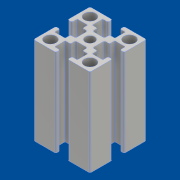
# Autodesk Inventor part: S31
Saved by Autodesk Inventor 2022.2 (Build 262287000, 287)
## iProperties
Created: 2018-10-03
Part Number: S31
Material: アルミニウム 6061
Document SubType Name: Modeling
Designer: gisen
Density: 2.7 g/cm^3
Appearance: アルミニウム - フラット
Author: gisen
Autodesk Inventor part; units mm, degrees
ref_plane "YZ Plane" through (0, 0, 0) normal (1, 0, 0) x (0, 1, 0)
ref_plane "XZ Plane" through (0, 0, 0) normal (0, 1, 0) x (-1, 0, 0)
ref_plane "XY Plane" through (0, 0, 0) normal (0, 0, 1) x (1, 0, 0)
sketch "BaseS" plane through (0, 0, 0) normal (0, 0, 1) x (1, 0, 0)
  line L0 (8.5, -3.8) -> (8.5, -2.6)
  line L1 (4, -8.3) -> (4, -5)
  circle A0 centre (7, -7) radius 2
  line L2 (10, -2.6) -> (10, -9.5)
  line L3 (2.6, -10) -> (9.5, -10)
  line L4 (2.1, -9.5) -> (2.1, -9)
  line L5 (8.5, -2.6) -> (8.5, -3.8)
  line L6 (3.8, -4.8) -> (2.6, -4.8)
  line L7 (4.8, -3.8) -> (4.8, -2.6)
  arc A1 (2.1, -4.3) -> (2.6, -4.8) centre (2.6, -4.3) ccw
  arc A2 (2.6, -8.5) -> (2.1, -9) centre (2.6, -9) ccw
  arc A3 (3.8, -8.5) -> (4, -8.3) centre (3.8, -8.3) ccw
  arc A4 (4, -5) -> (3.8, -4.8) centre (3.8, -5) ccw
  arc A5 (2.1, -3.5) -> (1.6, -3) centre (1.6, -3.5) ccw
  arc A6 (2.1, -9.5) -> (2.6, -10) centre (2.6, -9.5) ccw
  arc A7 (9.5, -10) -> (10, -9.5) centre (9.5, -9.5) ccw
  arc A8 (10, -2.6) -> (9.5, -2.1) centre (9.5, -2.6) ccw
  arc A9 (9, -2.1) -> (8.5, -2.6) centre (9, -2.6) ccw
  arc A10 (8.3, -4) -> (8.5, -3.8) centre (8.3, -3.8) ccw
  arc A11 (4.8, -3.8) -> (5, -4) centre (5, -3.8) ccw
  line L8 (4.3, -2.1) -> (3.5, -2.1)
  arc A12 (4.8, -2.6) -> (4.3, -2.1) centre (4.3, -2.6) ccw
  arc A13 (3, -1.6) -> (3.5, -2.1) centre (3.5, -1.6) ccw
  line L9 (2.1, -4.3) -> (2.1, -3.5)
  line L10 (3.8, -8.5) -> (2.6, -8.5)
  line L11 (9.5, -2.1) -> (9, -2.1)
  line L12 (8.3, -4) -> (5, -4)
  circle A14 centre (0, 0) radius 1.65
  arc A15 (8.5, 2.6) -> (9, 2.1) centre (9, 2.6) ccw
  line L13 (8.5, 3.8) -> (8.5, 2.6)
  arc A16 (8.5, 3.8) -> (8.3, 4) centre (8.3, 3.8) ccw
  line L14 (8.3, 4) -> (5, 4)
  line L15 (10, 2.6) -> (10, 9.5)
  arc A17 (10, 9.5) -> (9.5, 10) centre (9.5, 9.5) ccw
  circle A18 centre (7, 7) radius 2
  line L16 (4, 8.3) -> (4, 5)
  line L17 (2.6, 10) -> (9.5, 10)
  line L18 (9.5, 2.1) -> (9, 2.1)
  arc A19 (9.5, 2.1) -> (10, 2.6) centre (9.5, 2.6) ccw
  line L19 (3.8, 8.5) -> (2.6, 8.5)
  line L20 (4.8, 3.8) -> (4.8, 2.6)
  arc A20 (4.3, 2.1) -> (4.8, 2.6) centre (4.3, 2.6) ccw
  line L21 (2.6, 8.5) -> (3.8, 8.5)
  arc A21 (4, 8.3) -> (3.8, 8.5) centre (3.8, 8.3) ccw
  arc A22 (2.1, 9) -> (2.6, 8.5) centre (2.6, 9) ccw
  arc A23 (2.6, 10) -> (2.1, 9.5) centre (2.6, 9.5) ccw
  line L22 (2.1, 9.5) -> (2.1, 9)
  arc A24 (1.6, 3) -> (2.1, 3.5) centre (1.6, 3.5) ccw
  line L23 (3.8, 4.8) -> (2.6, 4.8)
  arc A25 (5, 4) -> (4.8, 3.8) centre (5, 3.8) ccw
  arc A26 (3.8, 4.8) -> (4, 5) centre (3.8, 5) ccw
  line L24 (4.3, 2.1) -> (3.5, 2.1)
  arc A27 (2.6, 4.8) -> (2.1, 4.3) centre (2.6, 4.3) ccw
  line L25 (2.1, 4.3) -> (2.1, 3.5)
  arc A28 (3.5, 2.1) -> (3, 1.6) centre (3.5, 1.6) ccw
  arc A29 (-2.6, 8.5) -> (-2.1, 9) centre (-2.6, 9) ccw
  line L26 (-3.8, 8.5) -> (-2.6, 8.5)
  arc A30 (-3.8, 8.5) -> (-4, 8.3) centre (-3.8, 8.3) ccw
  line L27 (-4, 8.3) -> (-4, 5)
  line L28 (-2.6, 10) -> (-9.5, 10)
  arc A31 (-9.5, 10) -> (-10, 9.5) centre (-9.5, 9.5) ccw
  circle A32 centre (-7, 7) radius 2
  line L29 (-8.3, 4) -> (-5, 4)
  line L30 (-10, 2.6) -> (-10, 9.5)
  line L31 (-2.1, 9.5) -> (-2.1, 9)
  arc A33 (-2.1, 9.5) -> (-2.6, 10) centre (-2.6, 9.5) ccw
  line L32 (-8.5, 3.8) -> (-8.5, 2.6)
  line L33 (-3.8, 4.8) -> (-2.6, 4.8)
  arc A34 (-2.1, 4.3) -> (-2.6, 4.8) centre (-2.6, 4.3) ccw
  line L34 (-8.5, 2.6) -> (-8.5, 3.8)
  arc A35 (-8.3, 4) -> (-8.5, 3.8) centre (-8.3, 3.8) ccw
  arc A36 (-9, 2.1) -> (-8.5, 2.6) centre (-9, 2.6) ccw
  arc A37 (-10, 2.6) -> (-9.5, 2.1) centre (-9.5, 2.6) ccw
  line L35 (-9.5, 2.1) -> (-9, 2.1)
  arc A38 (-3, 1.6) -> (-3.5, 2.1) centre (-3.5, 1.6) ccw
  line L36 (-4.8, 3.8) -> (-4.8, 2.6)
  arc A39 (-4, 5) -> (-3.8, 4.8) centre (-3.8, 5) ccw
  arc A40 (-4.8, 3.8) -> (-5, 4) centre (-5, 3.8) ccw
  line L37 (-2.1, 4.3) -> (-2.1, 3.5)
  arc A41 (-4.8, 2.6) -> (-4.3, 2.1) centre (-4.3, 2.6) ccw
  line L38 (-4.3, 2.1) -> (-3.5, 2.1)
  arc A42 (-2.1, 3.5) -> (-1.6, 3) centre (-1.6, 3.5) ccw
  arc A43 (-8.5, -2.6) -> (-9, -2.1) centre (-9, -2.6) ccw
  line L39 (-8.5, -3.8) -> (-8.5, -2.6)
  arc A44 (-8.5, -3.8) -> (-8.3, -4) centre (-8.3, -3.8) ccw
  line L40 (-8.3, -4) -> (-5, -4)
  line L41 (-10, -2.6) -> (-10, -9.5)
  arc A45 (-10, -9.5) -> (-9.5, -10) centre (-9.5, -9.5) ccw
  circle A46 centre (-7, -7) radius 2
  line L42 (-4, -8.3) -> (-4, -5)
  line L43 (-2.6, -10) -> (-9.5, -10)
  line L44 (-9.5, -2.1) -> (-9, -2.1)
  arc A47 (-9.5, -2.1) -> (-10, -2.6) centre (-9.5, -2.6) ccw
  line L45 (-3.8, -8.5) -> (-2.6, -8.5)
  line L46 (-4.8, -3.8) -> (-4.8, -2.6)
  arc A48 (-4.3, -2.1) -> (-4.8, -2.6) centre (-4.3, -2.6) ccw
  line L47 (-2.6, -8.5) -> (-3.8, -8.5)
  arc A49 (-4, -8.3) -> (-3.8, -8.5) centre (-3.8, -8.3) ccw
  arc A50 (-2.1, -9) -> (-2.6, -8.5) centre (-2.6, -9) ccw
  arc A51 (-2.6, -10) -> (-2.1, -9.5) centre (-2.6, -9.5) ccw
  line L48 (-2.1, -9.5) -> (-2.1, -9)
  arc A52 (-1.6, -3) -> (-2.1, -3.5) centre (-1.6, -3.5) ccw
  line L49 (-3.8, -4.8) -> (-2.6, -4.8)
  arc A53 (-5, -4) -> (-4.8, -3.8) centre (-5, -3.8) ccw
  arc A54 (-3.8, -4.8) -> (-4, -5) centre (-3.8, -5) ccw
  line L50 (-4.3, -2.1) -> (-3.5, -2.1)
  arc A55 (-2.6, -4.8) -> (-2.1, -4.3) centre (-2.6, -4.3) ccw
  line L51 (-2.1, -4.3) -> (-2.1, -3.5)
  arc A56 (-3.5, -2.1) -> (-3, -1.6) centre (-3.5, -1.6) ccw
  line L52 (1.6, -3) -> (-1.6, -3)
  line L53 (-3, -1.6) -> (-3, 1.6)
  line L54 (-1.6, 3) -> (1.6, 3)
  line L55 (3, 1.6) -> (3, -1.6)
  point P0 (2.1, -10)
  point P1 (10, 2.1)
  point P2 (-2.1, 10)
  point P3 (-10, -2.1)
  dimension "d2" = 4
  dimension "d3" = 3.7
  dimension "d4" = 0.5
  dimension "d5" = 0.5
  dimension "d6" = 0.2
  dimension "d7" = 0.5
  dimension "d8" = 0.5
  dimension "d9" = 0.5
  dimension "d10" = 0.2
  dimension "d11" = 0.5
  dimension "d12" = 1.5
  dimension "d13" = 3.7
  dimension "d14" = 1.5
  dimension "d15" = 3.3
  dimension "d16" = 10
  dimension "d17" = 2.1
  dimension "d18" = 2.1
  dimension "d19" = 1.9
  dimension "d20" = 7
  dimension "d21" = 2.1
  dimension "d22" = 2.1
  dimension "d23" = 1.9
  dimension "d24" = 7
  dimension "d25" = 10
  dimension "d26" = 360
  dimension "d27" = 3
  constraints: 112 end point, 104 point on circle, 57 centre point, 26 tangent, 20 point on line, 5 coincident, 5 equal radius, 5 horizontal, 4 vertical, 3 perpendicular, 281 other
  measures "d2" diameter of A0
  measures "d3" distance between parallel lines of L7 L0
  measures "d4" radius of A1
  measures "d5" radius of A2
  measures "d6" radius of A3
  measures "d7" radius of A5
  measures "d8" radius of A6
  measures "d9" radius of A7
  measures "d10" radius of A10
  measures "d11" radius of A12
  measures "d12" distance between parallel lines of L0 L2
  measures "d13" distance between parallel lines of L6 L10
  measures "d14" distance between parallel lines of L10 L3
  measures "d15" diameter of A14
  measures "d16" distance from line of L2 point (0, 0)
  measures "d17" distance from line of L9 point (0, 0)
  measures "d18" distance from line of L4 point (0, 0)
  measures "d19" distance between parallel lines of L1 L4
  measures "d20" horizontal distance of A0.centre point (0, 0)
  measures "d21" distance from line of L8 point (0, 0)
  measures "d22" distance from line of L11 point (0, 0)
  measures "d23" distance between parallel lines of L11 L12
  measures "d24" horizontal distance of A0.centre point (0, 0)
  measures "d25" distance from line of L3 point (0, 0)
  measures "d27" distance from line of L52 point (0, 0)
extrude "押し出し1" add sketch "BaseS" along normal blind 31
